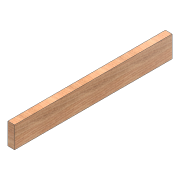
# Autodesk Inventor part: UprightStand_Back
Saved by Autodesk Inventor 2017 (Build 210142000, 142)
## iProperties
Created: 2017-05-22
Part Number: UprightStand_Back
Material: Generic
Document SubType Name: Modeling
Designer: krosie
Density: 1 g/cm^3
Appearance: Birch - Natural Polished
Author: krosie
Autodesk Inventor part; units mm, degrees
ref_plane "YZ Plane" through (0, 0, 0) normal (1, 0, 0) x (0, 1, 0)
ref_plane "XZ Plane" through (0, 0, 0) normal (0, 1, 0) x (-1, 0, 0)
ref_plane "XY Plane" through (0, 0, 0) normal (0, 0, 1) x (1, 0, 0)
sketch "Sketch1" plane through (0, 0, 0) normal (1, 0, 0) x (0, 1, 0)
  line L0 (-400, 55) -> (400, 55)
  line L1 (400, 55) -> (400, -55)
  line L2 (400, -55) -> (-400, -55)
  line L3 (-400, -55) -> (-400, 55)
  line L4 (-400, 55) -> (400, -55) construction
  line L5 (400, 55) -> (-400, -55) construction
  point P0 (0, 0)
  dimension "d0" = 800
  dimension "d1" = 110
  constraints: 12 end point, 2 midpoint, 2 parallel, 1 horizontal, 1 perpendicular
  measures "d0" distance of L1.end L2.end
  measures "d1" distance of L0.end L1.end
extrude "Extrusion1" add sketch "Sketch1" along normal blind 34
body "Solid1"
